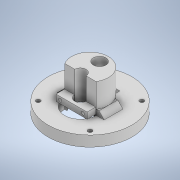
# Autodesk Inventor part: small_actuator_holder
Saved by Autodesk Inventor 2021 (Build 250183000, 183)
## iProperties
Created: 2020-10-24
Part Number: small_actuator_holder
Material: Generic
Document SubType Name: Modeling
Designer: bober
Density: 1 g/cm^3
Appearance: Default
Author: bober
Autodesk Inventor part; units mm, degrees
ref_plane "YZ Plane" through (0, 0, 0) normal (1, 0, 0) x (0, 1, 0)
ref_plane "XZ Plane" through (0, 0, 0) normal (0, 1, 0) x (-1, 0, 0)
ref_plane "XY Plane" through (0, 0, 0) normal (0, 0, 1) x (1, 0, 0)
sketch "Sketch1" plane through (0, 0, 0) normal (0, 1, 0) x (-1, 0, 0)
  circle A0 centre (0, 0) radius 17.5
  line L0 (-9.1924, 0) -> (0, 9.1924)
  line L1 (0, 9.1924) -> (9.1924, 0)
  line L2 (9.1924, 0) -> (0, -9.1924)
  line L3 (0, -9.1924) -> (-9.1924, 0)
  line L4 (-6.5, 6.5) -> (6.5, -6.5) construction
  line L5 (6.5, 6.5) -> (-6.5, -6.5) construction
  circle A1 centre (0, 9.1924) radius 5.45
  circle A2 centre (0, -9.1924) radius 6.025
  line L6 (-18.2848, 9.2924) -> (18.2848, 9.2924)
  line L7 (18.2848, 9.2924) -> (18.2848, 9.0924)
  line L8 (18.2848, 9.0924) -> (-18.2848, 9.0924)
  line L9 (-18.2848, 9.0924) -> (-18.2848, 9.2924)
  line L10 (-18.2848, 9.2924) -> (18.2848, 9.0924) construction
  line L11 (18.2848, 9.2924) -> (-18.2848, 9.0924) construction
  point P0 (5.4491, 9.2924)
  point P1 (14.8291, 9.2924)
  point P2 (-14.8291, 9.2924)
  point P3 (-5.4491, 9.2924)
  point P4 (-5.4491, 9.0924)
  point P5 (-14.9525, 9.0924)
  point P6 (14.9525, 9.0924)
  point P7 (5.4491, 9.0924)
  dimension "d0" = 35
  dimension "d1" = 13
  dimension "d2" = 13
  dimension "d3" = 10.9
  dimension "d4" = 12.05
  dimension "d5" = 0.2
  constraints: 24 end point, 4 midpoint, 4 parallel, 3 centre point, 3 coincident, 2 perpendicular, 1 horizontal
  measures "d0" diameter of A0
  measures "d1" distance of L1.end L2.end
  measures "d2" distance of L0.end L1.end
  measures "d3" diameter of A1
  measures "d4" diameter of A2
  measures "d5" distance of L6.end L7.end
extrude "Extrusion1" add sketch "Sketch1" along normal blind 29 contours A0 L8 A1 L0 L3 A2 L2 L1 | L6 A1 A0 | L1 L2 A2 L3 L0 A1
ref_plane "Work Plane1" through (5.4491, 0, -5.9076) normal (0, 0, 1) x (1, 0, 0)
sketch "Sketch4" plane through (5.4491, 0, -5.9076) normal (0, 0, 1) x (1, 0, 0)
  circle A0 centre (5.38, 5) radius 1.5 projected
  circle A1 centre (5.38, 5) radius 2.75
  line L0 (2.63, 6.5877) -> (5.38, 8.1754)
  line L1 (5.38, 8.1754) -> (8.13, 6.5877)
  line L2 (8.13, 6.5877) -> (8.13, 3.4123)
  line L3 (8.13, 3.4123) -> (5.38, 1.8246)
  line L4 (5.38, 1.8246) -> (2.63, 3.4123)
  line L5 (2.63, 3.4123) -> (2.63, 6.5877)
  circle A2 centre (5.38, 5) radius 2.75
  point P0 (-5.4491, 0)
  point P1 (2.63, 5)
  dimension "d17" = 5.5
  constraints: 12 end point, 2 coincident, 1 centre point, 1 horizontal alignment, 1 midpoint, 15 other
extrude "Extrusion2" cut sketch "Sketch4" against normal blind 19 contours A0 | A1 | L2 L3 A1 | A1 L1 L2 | A1 L0 L1 | L3 L4 A1 | A1 L5 L0 | L4 L5 A1
mirror "Mirror1" about plane through (0, 0, 0) normal (1, 0, 0) of "Extrusion2"
ref_plane "Work Plane2" through (5.4491, 0, 9.0924) normal (0, 0, 1) x (1, 0, 0)
ref_plane "Work Plane3" through (5.4491, 0, 12.0924) normal (0, 0, 1) x (1, 0, 0)
thicken "Thicken4" operation add thickness 5 both sides no extend neighbours yes toward (0, -1, 0) faces at (-8.6776, 0, 0.3947)
thicken "Thicken6" operation add thickness 4 both sides no extend neighbours yes toward (0, -1, 0) faces at (-8.6776, -5, 0.3947)
sketch "Sketch9" plane through (0, -9, 0) normal (0, -1, 0) x (1, 0, 0)
  circle A0 centre (0, 0) radius 17.5
  circle A1 centre (0, 0) radius 40
  arc A2 (-5.4491, 9.0924) -> (5.4491, 9.0924) centre (0, 9.1924) ccw projected
  circle A3 centre (0, 9.1924) radius 15
  point P0 (14.999, 9.0156)
  point P1 (-14.999, 9.0156)
  dimension "d48" = 35
  dimension "d49" = 80
  dimension "d50" = 30
  constraints: 3 centre point, 3 coincident
  measures "d48" diameter of A0
  measures "d49" diameter of A1
  measures "d50" diameter of A3
extrude "Extrusion5" add sketch "Sketch9" against normal blind 10
sketch "Sketch10" plane through (0, -9, 0) normal (0, -1, 0) x (1, 0, 0)
  circle A0 centre (-24.7487, 24.7487) radius 2
  point P0 (0, 0)
  dimension "d53" = 4
  constraints: 1 centre point
  measures "d53" diameter of A0
extrude "Extrusion6" cut sketch "Sketch10" against normal blind 10
pattern_circular "Circular Pattern1" count 4 over 360 about axis through (0, -9, 0) along (0, 1, 0) of "Extrusion6"
sketch "Sketch14" plane through (0, -9, 0) normal (0, -1, 0) x (1, 0, 0)
  circle A0 centre (0, 0) radius 15.6925
  dimension "d59" = 31.385
  constraints: 1 centre point, 1 coincident
  measures "d59" diameter of A0
extrude "Extrusion7" cut sketch "Sketch14" against normal blind 10
sketch "Sketch15" plane through (0, 1, 0) normal (0, 1, 0) x (1, 0, 0)
  line L0 (22.5, 9) -> (12.5, 9)
  line L1 (12.5, 9) -> (12.5, -9)
  line L2 (12.5, -9) -> (22.5, -9)
  line L3 (22.5, -9) -> (22.5, 9)
  arc A0 (14.9525, -9.0924) -> (-14.9525, -9.0924) centre (0, 0) ccw projected
  line L4 (22.5, 9) -> (12.5, -9) construction
  line L5 (12.5, 9) -> (22.5, -9) construction
  line L6 (-12.5, 9) -> (-22.5, 9)
  line L7 (-22.5, 9) -> (-22.5, -9)
  line L8 (-22.5, -9) -> (-12.5, -9)
  line L9 (-12.5, -9) -> (-12.5, 9)
  arc A1 (14.999, -9.0156) -> (-14.999, -9.0156) centre (0, 0) ccw projected
  line L10 (-12.5, 9) -> (-22.5, -9) construction
  line L11 (-22.5, 9) -> (-12.5, -9) construction
  line L12 (-6, 22.5) -> (6, 22.5)
  line L13 (6, 22.5) -> (6, 15.1924)
  line L14 (6, 15.1924) -> (-6, 15.1924)
  line L15 (-6, 15.1924) -> (-6, 22.5)
  point P0 (17.5, 0)
  point P1 (-17.5, 0)
  point P2 (-15.0083, -9)
  point P3 (-15.0083, 9)
  point P4 (-6, 16.4393)
  point P5 (6, 16.4393)
  point P6 (15.0083, 9)
  point P7 (15.0083, -9)
  dimension "d62" = 10
  dimension "d63" = 18
  dimension "d64" = 10
  dimension "d65" = 18
  dimension "d66" = 12
  constraints: 32 end point, 6 parallel, 4 midpoint, 3 horizontal, 3 perpendicular, 2 point on circle
  measures "d62" distance of L2.end L1.end
  measures "d63" distance of L1.end L0.end
  measures "d64" distance of L8.end L7.end
  measures "d65" distance of L7.end L6.end
  measures "d66" distance of L13.end L14.end
extrude "Extrusion8" add sketch "Sketch15" along normal blind 5 contours L3 L2 A0 L0 | A0 L15 L12 L13 | A0 L8 L7 L6
chamfer "Chamfer1" distance 5 angle 45 3 edges at (22.5, 6, 0) (0, 6, -22.5) (-22.5, 6, 0)
thicken "Thicken8" operation add thickness 1 both sides no extend neighbours yes toward (0, 1, 0) faces at (1.8681, 0, 16.1154)
thicken "Thicken9" operation add thickness 21 both sides no extend neighbours yes toward (0, -1, 0) faces at (10.8881, 29, 10.3158)
thicken "Thicken10" operation add thickness 1 both sides no extend neighbours yes toward (0, 1, 0) faces at (10.8881, 1, 10.3158)
sketch "Sketch17" plane through (14.8291, 8, 9.2924) normal (0, 0, -1) x (-1, 0, 0)
  line L0 (29.6582, 0) -> (0, 0) projected
  line L1 (9.38, -6) -> (9.38, 0) projected
  line L2 (0, 0) -> (9.38, 0)
  line L3 (9.38, 0) -> (9.38, -6)
  line L4 (9.38, -6) -> (0, -6)
  line L5 (0, -6) -> (0, 0)
  line L6 (20.2782, 0) -> (29.6582, 0) projected
  line L7 (29.6582, -6) -> (29.6582, 0) projected
  line L8 (20.2782, 0) -> (29.6582, 0)
  line L9 (29.6582, 0) -> (29.6582, -6)
  line L10 (29.6582, -6) -> (20.2782, -6)
  line L11 (20.2782, -6) -> (20.2782, 0)
  point P0 (14.8291, -8)
  constraints: 16 end point, 4 parallel, 2 horizontal, 2 perpendicular
extrude "Extrusion10" add sketch "Sketch17" against normal blind 7.3
sketch "Sketch18" plane through (14.8291, 8, 16.5924) normal (0, 0, 1) x (1, 0, 0)
  line L0 (0, -6) -> (-9.38, -6) projected
  line L1 (-20.2782, 0) -> (-29.6582, 0) projected
  line L2 (0, -6) -> (-29.6582, -6)
  line L3 (-29.6582, -6) -> (-29.6582, 0)
  line L4 (-29.6582, 0) -> (0, 0)
  line L5 (0, 0) -> (0, -6)
  point P0 (-14.8291, -8)
  constraints: 8 end point, 2 parallel, 1 horizontal, 1 perpendicular
extrude "Extrusion11" add sketch "Sketch18" along normal blind 1
sketch "Sketch16" plane through (5.4491, 29, 9.0924) normal (0, 0, 1) x (1, 0, 0)
  circle A0 centre (5.38, -24) radius 1.5
  circle A1 centre (-16.2782, -24) radius 1.5
  point P0 (-5.4491, -29)
  dimension "d75" = 3
  dimension "d76" = 3
  constraints: 2 centre point
  measures "d75" diameter of A0
  measures "d76" diameter of A1
extrude "Extrusion9" cut sketch "Sketch16" against normal mid plane 50
body "Solid1"
body "Solid6"
